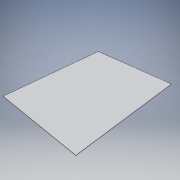
# Autodesk Inventor part: Baseplate
Saved by Autodesk Inventor 2019 (Build 230136000, 136)
## iProperties
Created: 2018-09-27
Part Number: Baseplate
Material: ABS Plastic
Document SubType Name: Modeling
Designer: Adhik
Density: 1.06 g/cm^3
Appearance: Smooth - White
Mass: 243.184 g
Surface Area: 2914.51 cm^2
Volume: 229.419 cm^3
Author: Adhik
Autodesk Inventor part; units mm, degrees
ref_plane "YZ Plane" through (0, 0, 0) normal (1, 0, 0) x (0, 1, 0)
ref_plane "XZ Plane" through (0, 0, 0) normal (0, 1, 0) x (-1, 0, 0)
ref_plane "XY Plane" through (0, 0, 0) normal (0, 0, 1) x (1, 0, 0)
sketch "Sketch1" plane through (0, 0, 0) normal (0, 1, 0) x (-1, 0, 0)
  line L0 (0, -320.04) -> (0, 320.04) construction
  line L1 (248.92, 0) -> (-248.92, 0) construction
  line L2 (177.8, -228.6) -> (-177.8, -228.6)
  line L3 (-177.8, -228.6) -> (-177.8, 228.6)
  line L4 (-177.8, 228.6) -> (177.8, 228.6)
  line L5 (177.8, 228.6) -> (177.8, -228.6)
  point P0 (0, 0)
  point P1 (177.8, 0)
  point P2 (0, -228.6)
  dimension "d0" = 355.6
  dimension "d1" = 457.2
  constraints: 8 end point, 2 midpoint, 2 parallel, 2 point on line, 1 horizontal, 1 perpendicular
  measures "d0" distance of L2.start L2.end
  measures "d1" distance of L4.end L2.start
extrude "Extrusion1" add sketch "Sketch1" along normal blind 1.5875
body "Solid1"
